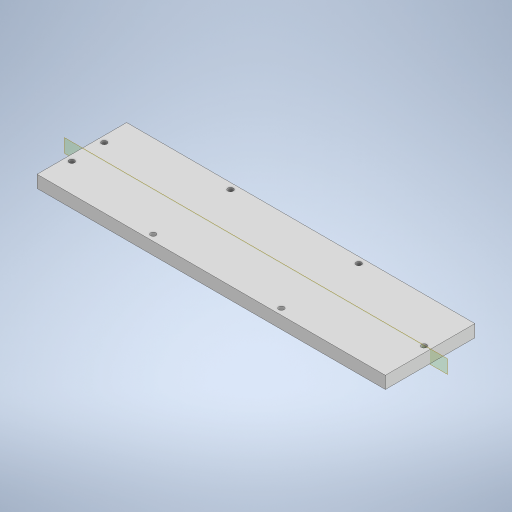
# Autodesk Inventor part: Mold_BottomWall
Saved by Autodesk Inventor 2024 (Build 280153000, 153)
## iProperties
Created: 2024-09-09
Part Number: Mold_BottomWall
Material: Generic
Document SubType Name: Modeling
Designer: Bruger
Density: 1 g/cm^3
Appearance: Default
Author: Bruger
Autodesk Inventor part; units mm, degrees
ref_plane "YZ Plane" through (0, 0, 0) normal (1, 0, 0) x (0, 1, 0)
ref_plane "XZ Plane" through (0, 0, 0) normal (0, 1, 0) x (-1, 0, 0)
sketch "Sketch1" plane through (0, 0, 0) normal (0, 1, 0) x (-1, 0, 0)
  line L0 (-72.97, 25.1) -> (125.33, 25.1)
  line L1 (125.33, 25.1) -> (125.33, -25.9)
  line L2 (125.33, -25.9) -> (-72.97, -25.9)
  line L3 (-72.97, -25.9) -> (-72.97, 25.1)
  line L4 (-72.97, 25.1) -> (125.33, -25.9) construction
  line L5 (125.33, 25.1) -> (-72.97, -25.9) construction
  point P0 (26.18, -0.4)
  dimension "d1" = 51
  dimension "d31" = 198.3
  constraints: 12 end point, 2 midpoint, 2 parallel, 1 horizontal, 1 perpendicular
  measures "d1" distance of L0.end L1.end
  measures "d31" distance of L1.end L2.end
extrude "Extrusion1" add sketch "Sketch1" along normal blind 7
sketch "Sketch2" plane through (0, 7, 0) normal (0, 1, 0) x (1, 0, 0)
  circle A0 centre (-121.83, 9.65) radius 1.5
  circle A1 centre (-62.665, 22.4) radius 1.5
  line L0 (72.97, 25.9) -> (-125.33, 25.9) projected
  line L1 (-125.33, 25.9) -> (-125.33, -25.1) projected
  circle A2 centre (69.47, 0.4) radius 1.5
  line L2 (72.97, -25.1) -> (72.97, 25.9) projected
  point P0 (0, 0)
  dimension "d5" = 3
  dimension "d21" = 3
  dimension "d22" = 3.5
  dimension "d23" = 62.665
  dimension "d32" = 3.5
  dimension "d33" = 16.25
  dimension "d34" = 3
  dimension "d35" = 3.5
  dimension "d36" = 25.5
  constraints: 3 centre point
  measures "d5" diameter of A0
  measures "d21" diameter of A1
  measures "d22" distance from line of L0 A1.centre
  measures "d23" distance from line of L1 A1.centre
  measures "d32" distance from line of L1 A0.centre
  measures "d33" distance from line of L0 A0.centre
  measures "d34" diameter of A2
  measures "d35" distance from line of L2 A2.centre
  measures "d36" distance from line of L0 A2.centre
hole "Hole1" at (-121.83, 7, -9.65) direction (0, -1, 0) diameter 3 end through all
hole "Hole3" at (-62.665, 7, -22.4) direction (0, -1, 0) diameter 3 end through all
ref_plane "Work Plane1" through (-26.18, 0, 25.1) normal (1, 0, 0) x (0, 0, -1)
mirror "Mirror7" about plane through (-26.18, 0, 25.1) normal (1, 0, 0) of "Hole3"
hole "Hole4" at (69.47, 7, -0.4) direction (0, -1, 0) diameter 3 end through all
ref_plane "Work Plane2" through (72.97, 0, -0.4) normal (0, 0, -1) x (-1, 0, 0)
mirror "Mirror8" about plane through (72.97, 0, -0.4) normal (0, 0, -1) of "Hole3", "Mirror7", "Hole1"
body "Solid1"
